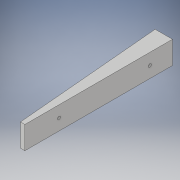
# Autodesk Inventor part: jigForRipCuts
Saved by Autodesk Inventor 2019.1 (Build 231200000, 200)
## iProperties
Created: 2018-07-31
Part Number: jigForRipCuts
Material: Generic
Document SubType Name: Modeling
Designer: steele
Density: 1 g/cm^3
Appearance: Default
Author: steele
Autodesk Inventor part; units mm, degrees
ref_plane "YZ Plane" through (0, 0, 0) normal (1, 0, 0) x (0, 1, 0)
ref_plane "XZ Plane" through (0, 0, 0) normal (0, 1, 0) x (-1, 0, 0)
sketch "Sketch1" plane through (0, 0, 0) normal (0, 1, 0) x (-1, 0, 0)
  line L0 (0, 0) -> (0, -330.2)
  line L1 (0, -330.2) -> (0, -122.0086)
  line L2 (0, -330.2) -> (28.8888, -330.2)
  line L3 (28.8888, -330.2) -> (0, 0)
  dimension "d0" = 330.2
  dimension "d1" = 5
  constraints: 8 end point, 1 horizontal, 1 point on line, 1 vertical
  measures "d0" distance of L0.start L0.end
  measures "d1" angle of L3 L0
extrude "Extrusion1" add sketch "Sketch1" along normal blind 50.8
ref_plane "Work Plane1" through (-28.8888, 50.8, -330.2) normal (1, 0, 0) x (0, 0, -1)
sketch "Sketch2" plane through (0, 0, 0) normal (1, 0, 0) x (0, 0, -1)
  line L0 (0, 0) -> (330.2, 0) projected
  line L1 (0, 50.8) -> (330.2, 50.8) projected
  line L2 (0, 0) -> (330.2, 0)
  line L3 (330.2, 0) -> (330.2, 50.8)
  line L4 (330.2, 50.8) -> (0, 50.8)
  line L5 (0, 50.8) -> (0, 0)
  constraints: 8 end point, 2 parallel, 1 horizontal, 1 perpendicular
extrude "Extrusion2" add sketch "Sketch2" along normal blind 9.8552
sketch "Sketch4" plane through (-28.8888, 50.8, -330.2) normal (1, 0, 0) x (0, 0, -1)
  line L0 (0, -50.8) -> (0, 0) construction
  line L1 (0, -25.4) -> (-279.4, -25.4) construction
  line L2 (0, -50.8) -> (-330.2, -50.8) construction
  line L3 (-330.2, -50.8) -> (-330.2, 0) construction
  point P0 (-254, -25.4)
  point P1 (-50.8, -25.4)
  point P2 (-330.2, 0)
  dimension "d16" = 25.4
  dimension "d17" = 76.2
  dimension "d18" = 279.4
  constraints: 2 end point, 2 point on line, 1 horizontal, 1 midpoint, 1 other
  measures "d16" distance between parallel lines of L1 L2
hole "Hole2" at (-28.8888, 25.4, -76.2) at (-28.8888, 25.4, -279.4) direction (1, 0, 0) diameter 6.7564 end through all counterbore diameter 17.78 counterbore depth 27.94 clearance for "Socket Head Cap Screw" size "1/4" standard "Ansi Unified Screw Threads"
equation "\"d0\" = lengthOfFixture"
equation "\"d1\" = cutAngle"
equation "\"d2\" = heightOfJig"
equation "\"d4\" = addedDepthToSupportBolts"
equation "\"d16\" = heightOfBoltHolt"
equation "\"d17\" = bottomToFirstHole"
equation "\"d18\" = bottomToSecondHole"
equation "\"lengthOfFixture\" = 330.2"
equation "\"cutAngle\" = 5deg"
equation "\"bottomToFirstHole\" = 76.2"
equation "\"distanceBetweenBolts\" = 203.2"
equation "\"bottomToSecondHole\" = bottomToFirstHole + distanceBetweenBolts"
equation "\"heightOfBoltHolt\" = 25.4"
equation "\"boltSize\" = 6.35"
equation "\"heightOfJig\" = 50.8"
equation "\"addedDepthToSupportBolts\" = 9.8552"
body "Solid1"
